Autodesk Fusion 360 part; units mm, degrees
note: some values were not read from the file. Chosen so that the rebuilt part matches the saved one: which bodies a step acts on; which sketch regions a step uses.
(part 6 of 6)
  line L3303 (-33.1167, -64.6164) -> (-31.8667, -62.4513)
  line L3304 (-48.2879, -61.8648) -> (-47.0379, -59.6997)
  line L3305 (-92.6, -56.7847) -> (-93.85, -54.6196)
  line L3306 (-20.4213, -63.2013) -> (-21.6713, -65.3664)
  line L3307 (-36.8667, -62.4513) -> (-35.6167, -64.6164)
  line L3308 (-60.9101, -61.8648) -> (-58.4101, -61.8648)
  line L3309 (-46.9889, -62.4513) -> (-45.7389, -64.6164)
  line L3310 (-35.6167, -60.2863) -> (-36.8667, -62.4513)
  line L3311 (-58.4101, -61.8648) -> (-57.1601, -59.6997)
  line L3312 (-45.7389, -64.6164) -> (-43.2389, -64.6164)
  line L3313 (-22.9944, -64.6164) -> (-21.7444, -62.4513)
  line L3314 (-30.5435, -63.2013) -> (-31.7935, -65.3664)
  line L3315 (-10.299, -63.2013) -> (-11.549, -65.3664)
  line L3316 (-58.4101, -57.5347) -> (-60.9101, -57.5347)
  line L3317 (-50.7879, -67.5315) -> (-48.2879, -67.5315)
  line L3318 (-101.399, -61.8648) -> (-98.899, -61.8648)
  line L3319 (-43.2389, -60.2863) -> (-45.7389, -60.2863)
  line L3320 (-12.8722, -64.6164) -> (-11.6222, -62.4513)
  line L3321 (-10.299, -67.5315) -> (-7.799, -67.5315)
  line L3322 (-91.2768, -61.8648) -> (-88.7768, -61.8648)
  line L3323 (-7.799, -67.5315) -> (-6.549, -65.3664)
  line L3324 (-52.0379, -65.3664) -> (-50.7879, -67.5315)
  line L3325 (-21.7444, -62.4513) -> (-22.9944, -60.2863)
  line L3326 (-26.7935, -65.3664) -> (-28.0435, -63.2013)
  line L3327 (-5.25, -64.6164) -> (-2.75, -64.6164)
  line L3328 (-20.4213, -67.5315) -> (-17.9213, -67.5315)
  line L3329 (-25.4944, -60.2863) -> (-26.7444, -62.4513)
  line L3330 (-68.5324, -57.5347) -> (-71.0324, -57.5347)
  line L3331 (-38.1657, -63.2013) -> (-40.6657, -63.2013)
  line L3332 (-1.5, -62.4513) -> (-2.75, -60.2863)
  line L3333 (-48.2879, -63.2013) -> (-50.7879, -63.2013)
  line L3334 (-43.2389, -64.6164) -> (-41.9889, -62.4513)
  line L3335 (-98.899, -61.8648) -> (-97.649, -59.6997)
  line L3336 (-6.5, -62.4513) -> (-5.25, -64.6164)
  line L3337 (-45.7389, -60.2863) -> (-46.9889, -62.4513)
  line L3338 (-30.5435, -67.5315) -> (-28.0435, -67.5315)
  line L3339 (-22.9944, -60.2863) -> (-25.4944, -60.2863)
  line L3340 (-11.6222, -62.4513) -> (-12.8722, -60.2863)
  line L3341 (-6.549, -65.3664) -> (-7.799, -63.2013)
  line L3342 (-98.899, -57.5347) -> (-101.399, -57.5347)
  line L3343 (-33.1167, -60.2863) -> (-35.6167, -60.2863)
  line L3344 (-78.6546, -61.8648) -> (-77.4046, -59.6997)
  line L3345 (-96.35, -58.9497) -> (-93.85, -58.9497)
  line L3346 (-57.1111, -56.7847) -> (-55.8611, -58.9497)
  line L3347 (-28.0435, -63.2013) -> (-30.5435, -63.2013)
  line L3348 (-97.649, -59.6997) -> (-98.899, -57.5347)
  line L3349 (-63.4833, -58.9497) -> (-62.2333, -56.7847)
  line L3350 (-41.9157, -65.3664) -> (-40.6657, -67.5315)
  line L3351 (-40.6657, -67.5315) -> (-38.1657, -67.5315)
  line L3352 (-17.9213, -67.5315) -> (-16.6713, -65.3664)
  line L3353 (-26.7444, -62.4513) -> (-25.4944, -64.6164)
  line L3354 (-15.3722, -60.2863) -> (-16.6222, -62.4513)
  line L3355 (-96.35, -54.6196) -> (-97.6, -56.7847)
  line L3356 (-15.3722, -64.6164) -> (-12.8722, -64.6164)
  line L3357 (-31.7935, -65.3664) -> (-30.5435, -67.5315)
  line L3358 (-50.7879, -63.2013) -> (-52.0379, -65.3664)
  line L3359 (-11.549, -65.3664) -> (-10.299, -67.5315)
  line L3360 (-2.75, -60.2863) -> (-5.25, -60.2863)
  line L3361 (-52.1111, -62.4513) -> (-53.3611, -60.2863)
  line L3362 (-55.8611, -60.2863) -> (-57.1111, -62.4513)
  line L3363 (-60.9101, -67.5315) -> (-58.4101, -67.5315)
  line L3364 (-91.2768, -63.2013) -> (-92.5268, -65.3664)
  line L3365 (-78.6546, -67.5315) -> (-77.4046, -65.3664)
  line L3366 (-67.2824, -65.3664) -> (-68.5324, -63.2013)
  line L3367 (-73.6056, -60.2863) -> (-76.1056, -60.2863)
  line L3368 (-68.5324, -63.2013) -> (-71.0324, -63.2013)
  line L3369 (-82.4778, -62.4513) -> (-83.7278, -60.2863)
  line L3370 (-63.4833, -60.2863) -> (-65.9833, -60.2863)
  line L3371 (-53.3611, -60.2863) -> (-55.8611, -60.2863)
  line L3372 (-7.799, -63.2013) -> (-10.299, -63.2013)
  line L3373 (-2.75, -64.6164) -> (-1.5, -62.4513)
  line L3374 (-91.2768, -67.5315) -> (-88.7768, -67.5315)
  line L3375 (-63.4833, -64.6164) -> (-62.2333, -62.4513)
  line L3376 (-76.1056, -60.2863) -> (-77.3556, -62.4513)
  line L3377 (-78.6546, -63.2013) -> (-81.1546, -63.2013)
  line L3378 (-101.399, -57.5347) -> (-102.649, -59.6997)
  line L3379 (-92.5268, -65.3664) -> (-91.2768, -67.5315)
  line L3380 (-58.4101, -63.2013) -> (-60.9101, -63.2013)
  line L3381 (-12.8722, -60.2863) -> (-15.3722, -60.2863)
  line L3382 (-5.25, -60.2863) -> (-6.5, -62.4513)
  line L3383 (-68.5324, -67.5315) -> (-67.2824, -65.3664)
  line L3384 (-87.4778, -62.4513) -> (-86.2278, -64.6164)
  line L3385 (-67.2333, -62.4513) -> (-65.9833, -64.6164)
  line L3386 (-65.9833, -60.2863) -> (-67.2333, -62.4513)
  line L3387 (-58.4101, -67.5315) -> (-57.1601, -65.3664)
  line L3388 (-86.2278, -60.2863) -> (-87.4778, -62.4513)
  line L3389 (-55.8611, -64.6164) -> (-53.3611, -64.6164)
  line L3390 (-88.7768, -63.2013) -> (-91.2768, -63.2013)
  line L3391 (-77.3556, -62.4513) -> (-76.1056, -64.6164)
  line L3392 (-71.0324, -67.5315) -> (-68.5324, -67.5315)
  line L3393 (-77.3556, -11.4513) -> (-76.1056, -13.6164)
  line L3394 (-77.4046, -65.3664) -> (-78.6546, -63.2013)
  line L3395 (-17.9213, -63.2013) -> (-20.4213, -63.2013)
  line L3396 (-73.6056, -64.6164) -> (-72.3556, -62.4513)
  line L3397 (-76.1056, -13.6164) -> (-73.6056, -13.6164)
  line L3398 (-73.6056, -13.6164) -> (-72.3556, -11.4513)
  line L3399 (-38.1657, -67.5315) -> (-36.9157, -65.3664)
  line L3400 (-86.2278, -64.6164) -> (-83.7278, -64.6164)
  line L3401 (-88.7768, -67.5315) -> (-87.5268, -65.3664)
  line L3402 (-62.2333, -62.4513) -> (-63.4833, -60.2863)
  line L3403 (-62.1601, -65.3664) -> (-60.9101, -67.5315)
  line L3404 (-72.3556, -62.4513) -> (-73.6056, -60.2863)
  line L3405 (-81.1546, -63.2013) -> (-82.4046, -65.3664)
  line L3406 (-21.6713, -65.3664) -> (-20.4213, -67.5315)
  line L3407 (-76.1056, -64.6164) -> (-73.6056, -64.6164)
  line L3408 (-57.1601, -65.3664) -> (-58.4101, -63.2013)
  line L3409 (-40.6657, -63.2013) -> (-41.9157, -65.3664)
  line L3410 (-60.9101, -63.2013) -> (-62.1601, -65.3664)
  line L3411 (-72.2824, -65.3664) -> (-71.0324, -67.5315)
  line L3412 (-81.1546, -67.5315) -> (-78.6546, -67.5315)
  line L3413 (-65.9833, -64.6164) -> (-63.4833, -64.6164)
  line L3414 (-83.7278, -60.2863) -> (-86.2278, -60.2863)
  line L3415 (-71.0324, -63.2013) -> (-72.2824, -65.3664)
  line L3416 (-57.1111, -62.4513) -> (-55.8611, -64.6164)
  line L3417 (-28.0435, -67.5315) -> (-26.7935, -65.3664)
  line L3418 (-53.3611, -64.6164) -> (-52.1111, -62.4513)
  line L3419 (-48.2879, -67.5315) -> (-47.0379, -65.3664)
  line L3420 (-82.4046, -65.3664) -> (-81.1546, -67.5315)
  line L3421 (-41.9889, -62.4513) -> (-43.2389, -60.2863)
  line L3422 (-83.7278, -64.6164) -> (-82.4778, -62.4513)
  line L3423 (-47.0379, -65.3664) -> (-48.2879, -63.2013)
  line L3424 (-25.4944, -64.6164) -> (-22.9944, -64.6164)
  line L3425 (-72.3556, -11.4513) -> (-73.6056, -9.2863)
  line L3426 (-73.6056, -9.2863) -> (-76.1056, -9.2863)
  line L3427 (-86.2278, -13.6164) -> (-83.7278, -13.6164)
  line L3428 (-81.1546, -12.2013) -> (-82.4046, -14.3664)
  line L3429 (-82.4046, -14.3664) -> (-81.1546, -16.5315)
  line L3430 (-81.1546, -16.5315) -> (-78.6546, -16.5315)
  line L3431 (-77.4046, -14.3664) -> (-78.6546, -12.2013)
  line L3432 (-87.4778, -11.4513) -> (-86.2278, -13.6164)
  line L3433 (-76.1056, -9.2863) -> (-77.3556, -11.4513)
  line L3434 (-78.6546, -12.2013) -> (-81.1546, -12.2013)
  line L3435 (-78.6546, -16.5315) -> (-77.4046, -14.3664)
  line L3436 (-83.7278, -13.6164) -> (-82.4778, -11.4513)
  line L3437 (-82.4778, -11.4513) -> (-83.7278, -9.2863)
  line L3438 (-83.7278, -9.2863) -> (-86.2278, -9.2863)
  line L3439 (-100, -76.4513) -> (0, -76.4513)
  arc A0 (-83, -31.5) -> (-81.5, -30) centre (-81.5, -31.5) cw
  line L3440 (-5.25, -77.2863) -> (-6.5, -79.4513)
  line L3441 (-7.5, -67) -> (-8.5, -67)
  arc A1 (-81.5, -67.1954) -> (-83, -65.6954) centre (-81.5, -65.6954) cw
  line L3442 (-83.3, -46.9053) -> (-88.25, -49.7631)
  line L3443 (0, -21) -> (-100, -21)
  arc A2 (-90.5, -30) -> (-89, -31.5) centre (-90.5, -31.5) cw
  line L3444 (-100, -74.4513) -> (0, -74.4513)
  line L3445 (0, -74.4513) -> (0, -21)
  arc A3 (-94, -31.5) -> (-92.5, -30) centre (-92.5, -31.5) cw
  circle A4 centre (-50, -50) radius 3.175
  arc A5 (-89, -65.5) -> (-90.5, -67) centre (-90.5, -65.5) cw
  line L3446 (-81, -67.1954) -> (-81.5, -67.1954)
  line L3447 (-90.5, -67) -> (-92.5, -67)
  line L3448 (-94, -65.5) -> (-94, -31.5)
  arc A6 (-7.5, -30) -> (-6, -31.5) centre (-7.5, -31.5) cw
  arc A7 (-83, -47.0785) -> (-83.3, -46.9053) centre (-83.2, -47.0785) ccw
  arc A8 (-83.75, -45.433) -> (-83, -44.134) centre (-84.5, -44.134) ccw
  arc A9 (-81, -30) -> (-79.5, -31.5) centre (-81, -31.5) cw
  line L3449 (-89, -51.0622) -> (-89, -65.5)
  line L3450 (-89, -31.5) -> (-89, -48.1177)
  line L3451 (-79.5, -31.5) -> (-79.5, -65.6954)
  arc A10 (-79.5, -65.6954) -> (-81, -67.1954) centre (-81, -65.6954) cw
  arc A11 (-89, -48.1177) -> (-88.7, -48.2909) centre (-88.8, -48.1177) ccw
  line L3452 (-83, -65.6954) -> (-83, -47.0785)
  arc A12 (-88.25, -49.7631) -> (-89, -51.0622) centre (-87.5, -51.0622) ccw
  line L3453 (-10, -65.5) -> (-10, -31.5)
  line L3454 (-6, -31.5) -> (-6, -65.5)
  line L3455 (-6.5, -79.4513) -> (-5.25, -81.6164)
  line L3456 (-92.5, -30) -> (-90.5, -30)
  line L3457 (-81.5, -30) -> (-81, -30)
  line L3458 (-5.25, -81.6164) -> (-2.75, -81.6164)
  line L3459 (-2.75, -77.2863) -> (-5.25, -77.2863)
  line L3460 (-8.5, -30) -> (-7.5, -30)
  line L3461 (-83, -44.134) -> (-83, -31.5)
  line L3462 (-2.75, -81.6164) -> (-1.5, -79.4513)
  line L3463 (-88.7, -48.2909) -> (-83.75, -45.433)
  arc A13 (-92.5, -67) -> (-94, -65.5) centre (-92.5, -65.5) cw
  arc A14 (-8.5, -67) -> (-10, -65.5) centre (-8.5, -65.5) cw
  line L3464 (-6.549, -3.0331) -> (-7.799, -0.868)
  line L3465 (-100, -21) -> (-100, -74.4513)
  line L3466 (-1.5, -79.4513) -> (-2.75, -77.2863)
  line L3467 (-10.299, -80.2013) -> (-11.549, -82.3664)
  line L3468 (0, -76.4513) -> (0, -84.1184)
  line L3469 (-11.6222, -0.118) -> (-12.8722, 2.0471)
  line L3470 (-36.8667, -0.118) -> (-35.6167, -2.2831)
  line L3471 (-21.7444, -0.118) -> (-22.9944, 2.0471)
  line L3472 (-7.799, -80.2013) -> (-10.299, -80.2013)
  line L3473 (-21.6713, -3.0331) -> (-20.4213, -5.1981)
  line L3474 (-33.1167, 2.0471) -> (-35.6167, 2.0471)
  line L3475 (-2.75, 2.0471) -> (-5.25, 2.0471)
  line L3476 (-11.549, -82.3664) -> (-10.299, -84.5315)
  line L3477 (-45.7389, 2.0471) -> (-46.9889, -0.118)
  line L3478 (-50.7879, -0.868) -> (-52.0379, -3.0331)
  line L3479 (-33.1167, -2.2831) -> (-31.8667, -0.118)
  line L3480 (-17.9213, -0.868) -> (-20.4213, -0.868)
  line L3481 (-12.8722, -2.2831) -> (-11.6222, -0.118)
  line L3482 (-4, -79.4513) -> (-10.924, -83.4489)
  line L3483 (-5.25, -2.2831) -> (-2.75, -2.2831)
  line L3484 (-7.799, -84.5315) -> (-6.549, -82.3664)
  line L3485 (-20.4213, -5.1981) -> (-17.9213, -5.1981)
  line L3486 (-40.6657, -5.1981) -> (-38.1657, -5.1981)
  line L3487 (-41.9889, -0.118) -> (-43.2389, 2.0471)
  line L3488 (-31.8667, -0.118) -> (-33.1167, 2.0471)
  line L3489 (-6.549, -82.3664) -> (-7.799, -80.2013)
  line L3490 (-17.9213, -5.1981) -> (-16.6713, -3.0331)
  line L3491 (-28.0435, -5.1981) -> (-26.7935, -3.0331)
  line L3492 (-40.6657, -0.868) -> (-41.9157, -3.0331)
  arc A15 (-6, -65.5) -> (-7.5, -67) centre (-7.5, -65.5) cw
  line L3493 (-30.5435, -5.1981) -> (-28.0435, -5.1981)
  line L3494 (-26.7935, -3.0331) -> (-28.0435, -0.868)
  line L3495 (-43.2389, -2.2831) -> (-41.9889, -0.118)
  line L3496 (-16.6713, -3.0331) -> (-17.9213, -0.868)
  arc A16 (-10, -31.5) -> (-8.5, -30) centre (-8.5, -31.5) cw
  line L3497 (-43.2389, 2.0471) -> (-45.7389, 2.0471)
  line L3498 (-28.0435, -0.868) -> (-30.5435, -0.868)
  line L3499 (-5.25, 2.0471) -> (-6.5, -0.118)
  line L3500 (-41.9157, -3.0331) -> (-40.6657, -5.1981)
  line L3501 (-52.0379, -3.0331) -> (-50.7879, -5.1981)
  line L3502 (-31.7935, -3.0331) -> (-30.5435, -5.1981)
  line L3503 (-48.2879, -0.868) -> (-50.7879, -0.868)
  line L3504 (-50.7879, -5.1981) -> (-48.2879, -5.1981)
  line L3505 (-20.4213, -0.868) -> (-21.6713, -3.0331)
  line L3506 (-30.5435, -0.868) -> (-31.7935, -3.0331)
  line L3507 (-22.9944, -2.2831) -> (-21.7444, -0.118)
  line L3508 (-10.299, -5.1981) -> (-7.799, -5.1981)
  line L3509 (-45.7389, -2.2831) -> (-43.2389, -2.2831)
  line L3510 (-6.5, -0.118) -> (-5.25, -2.2831)
  line L3511 (-7.799, -5.1981) -> (-6.549, -3.0331)
  line L3512 (-2.75, -2.2831) -> (-1.5, -0.118)
  line L3513 (-26.7444, -0.118) -> (-25.4944, -2.2831)
  line L3514 (-15.3722, -2.2831) -> (-12.8722, -2.2831)
  line L3515 (-35.6167, 2.0471) -> (-36.8667, -0.118)
  line L3516 (-11.549, -3.0331) -> (-10.299, -5.1981)
  line L3517 (-15.3722, 2.0471) -> (-16.6222, -0.118)
  line L3518 (-73.6056, 2.0471) -> (-76.1056, 2.0471)
  line L3519 (-65.9833, -2.2831) -> (-63.4833, -2.2831)
  line L3520 (-25.4944, 2.0471) -> (-26.7444, -0.118)
  line L3521 (-86.2278, 2.0471) -> (-87.4778, -0.118)
  line L3522 (-72.2824, -3.0331) -> (-71.0324, -5.1981)
  line L3523 (-91.2768, -0.868) -> (-92.5268, -3.0331)
  line L3524 (-93.85, -2.2831) -> (-92.6, -0.118)
  line L3525 (-35.6167, -2.2831) -> (-33.1167, -2.2831)
  line L3526 (-46.9889, -0.118) -> (-45.7389, -2.2831)
  line L3527 (-38.1657, -5.1981) -> (-36.9157, -3.0331)
  line L3528 (-1.5, -0.118) -> (-2.75, 2.0471)
  line L3529 (-10.299, -84.5315) -> (-7.799, -84.5315)
  line L3530 (-55.8611, 2.0471) -> (-57.1111, -0.118)
  line L3531 (-92.6, -0.118) -> (-93.85, 2.0471)
  line L3532 (-96.35, 2.0471) -> (-97.6, -0.118)
  line L3533 (-38.1657, -0.868) -> (-40.6657, -0.868)
  line L3534 (-96.35, -2.2831) -> (-93.85, -2.2831)
  line L3535 (-12.8722, 2.0471) -> (-15.3722, 2.0471)
  line L3536 (-36.9157, -3.0331) -> (-38.1657, -0.868)
  line L3537 (-16.6222, -0.118) -> (-15.3722, -2.2831)
  line L3538 (-7.799, -0.868) -> (-10.299, -0.868)
  line L3539 (-71.0324, -5.1981) -> (-68.5324, -5.1981)
  line L3540 (-101.399, -0.868) -> (-102.649, -3.0331)
  line L3541 (-57.1601, -3.0331) -> (-58.4101, -0.868)
  line L3542 (-22.9944, 2.0471) -> (-25.4944, 2.0471)
  line L3543 (-10.299, -0.868) -> (-11.549, -3.0331)
  line L3544 (-25.4944, -2.2831) -> (-22.9944, -2.2831)
  line L3545 (-53.3611, -2.2831) -> (-52.1111, -0.118)
  line L3546 (-86.2278, -2.2831) -> (-83.7278, -2.2831)
  line L3547 (-77.3556, -0.118) -> (-76.1056, -2.2831)
  line L3548 (-67.2824, -3.0331) -> (-68.5324, -0.868)
  line L3549 (-71.0324, -0.868) -> (-72.2824, -3.0331)
  line L3550 (-48.2879, -5.1981) -> (-47.0379, -3.0331)
  line L3551 (-98.899, -5.1981) -> (-97.649, -3.0331)
  line L3552 (-83.7278, -2.2831) -> (-82.4778, -0.118)
  line L3553 (-102.649, -3.0331) -> (-101.399, -5.1981)
  line L3554 (-62.2333, -0.118) -> (-63.4833, 2.0471)
  line L3555 (-43.2389, -71.6196) -> (-45.7389, -71.6196)
  line L3556 (-45.7389, -71.6196) -> (-46.9889, -73.7847)
  line L3557 (-50.7879, -74.5347) -> (-52.0379, -76.6997)
  line L3558 (-48.2879, -74.5347) -> (-50.7879, -74.5347)
  line L3559 (-52.0379, -76.6997) -> (-50.7879, -78.8648)
  line L3560 (-45.7389, -65.9529) -> (-46.9889, -68.118)
  line L3561 (-43.2389, -65.9529) -> (-45.7389, -65.9529)
  line L3562 (-41.9889, -68.118) -> (-43.2389, -65.9529)
  line L3563 (-48.2879, -73.1981) -> (-47.0379, -71.0331)
  line L3564 (-50.7879, -73.1981) -> (-48.2879, -73.1981)
  line L3565 (-47.0379, -71.0331) -> (-48.2879, -68.868)
  line L3566 (-57.1111, -68.118) -> (-55.8611, -70.2831)
  line L3567 (-53.3611, -70.2831) -> (-52.1111, -68.118)
  line L3568 (-52.0379, -71.0331) -> (-50.7879, -73.1981)
  line L3569 (-50.7879, -78.8648) -> (-48.2879, -78.8648)
  line L3570 (-50.7879, -68.868) -> (-52.0379, -71.0331)
  line L3571 (-55.8611, -65.9529) -> (-57.1111, -68.118)
  line L3572 (-63.4833, -70.2831) -> (-62.2333, -68.118)
  line L3573 (-65.9833, -65.9529) -> (-67.2333, -68.118)
  line L3574 (-81.1546, -68.868) -> (-82.4046, -71.0331)
  line L3575 (-73.6056, -70.2831) -> (-72.3556, -68.118)
  line L3576 (-87.4778, -68.118) -> (-86.2278, -70.2831)
  line L3577 (-68.5324, -68.868) -> (-71.0324, -68.868)
  line L3578 (-58.4101, -68.868) -> (-60.9101, -68.868)
  line L3579 (-93.85, -70.2831) -> (-92.6, -68.118)
  line L3580 (-60.9101, -73.1981) -> (-58.4101, -73.1981)
  line L3581 (-68.5324, -73.1981) -> (-67.2824, -71.0331)
  line L3582 (-92.5268, -71.0331) -> (-91.2768, -73.1981)
  line L3583 (-76.1056, -70.2831) -> (-73.6056, -70.2831)
  line L3584 (-73.6056, -65.9529) -> (-76.1056, -65.9529)
  line L3585 (-92.6, -68.118) -> (-93.85, -65.9529)
  line L3586 (-72.3556, -68.118) -> (-73.6056, -65.9529)
  line L3587 (-58.4101, -73.1981) -> (-57.1601, -71.0331)
  line L3588 (-72.2824, -71.0331) -> (-71.0324, -73.1981)
  line L3589 (-86.2278, -70.2831) -> (-83.7278, -70.2831)
  line L3590 (-65.9833, -70.2831) -> (-63.4833, -70.2831)
  line L3591 (-62.1601, -71.0331) -> (-60.9101, -73.1981)
  line L3592 (-62.2333, -68.118) -> (-63.4833, -65.9529)
  line L3593 (-67.2824, -71.0331) -> (-68.5324, -68.868)
  line L3594 (-91.2768, -73.1981) -> (-88.7768, -73.1981)
  line L3595 (-76.1056, -65.9529) -> (-77.3556, -68.118)
  line L3596 (-52.1111, -68.118) -> (-53.3611, -65.9529)
  line L3597 (-83.7278, -70.2831) -> (-82.4778, -68.118)
  line L3598 (-83.7278, -65.9529) -> (-86.2278, -65.9529)
  line L3599 (-88.7768, -68.868) -> (-91.2768, -68.868)
  line L3600 (-96.35, -70.2831) -> (-93.85, -70.2831)
  line L3601 (-78.6546, -68.868) -> (-81.1546, -68.868)
  line L3602 (-91.2768, -68.868) -> (-92.5268, -71.0331)
  line L3603 (-93.85, -65.9529) -> (-96.35, -65.9529)
  line L3604 (-60.9101, -68.868) -> (-62.1601, -71.0331)
  line L3605 (-71.0324, -73.1981) -> (-68.5324, -73.1981)
  line L3606 (-82.4778, -68.118) -> (-83.7278, -65.9529)
  line L3607 (-77.4046, -71.0331) -> (-78.6546, -68.868)
  line L3608 (-55.8611, -70.2831) -> (-53.3611, -70.2831)
  line L3609 (-96.35, -65.9529) -> (-97.6, -68.118)
  line L3610 (-101.399, -68.868) -> (-102.649, -71.0331)
  line L3611 (-82.4046, -71.0331) -> (-81.1546, -73.1981)
  line L3612 (-67.2333, -68.118) -> (-65.9833, -70.2831)
  line L3613 (-63.4833, -65.9529) -> (-65.9833, -65.9529)
  line L3614 (-86.2278, -65.9529) -> (-87.4778, -68.118)
  line L3615 (-77.3556, -68.118) -> (-76.1056, -70.2831)
  line L3616 (-102.649, -71.0331) -> (-101.399, -73.1981)
  line L3617 (-71.0324, -68.868) -> (-72.2824, -71.0331)
  line L3618 (-48.2879, -68.868) -> (-50.7879, -68.868)
  line L3619 (-57.1601, -71.0331) -> (-58.4101, -68.868)
  line L3620 (-81.1546, -73.1981) -> (-78.6546, -73.1981)
  line L3621 (-78.6546, -73.1981) -> (-77.4046, -71.0331)
  line L3622 (-53.3611, -65.9529) -> (-55.8611, -65.9529)
extrude "Extrude22" cut sketch "holes" against normal up to surface (2.5 mm away) contours L0 L9 L26 L27 L40 L43 | L3 L10 L11 L33 L48 L54 | L4 L15 L28 L35 L55 L120 | L5 L6 L17 L39 L47 L123 | L12 L14 L25 L32 L42 L126 | L13 L16 L22 L31 L41 L45 | L19 L20 L21 L24 L121 L125 | L56 L73 L76 L83 L87 L1162 | L57 L60 L69 L77 L103 L109 | L59 L72 L84 L92 L104 L111 | L63 L64 L78 L90 L105 L113 | L70 L85 L88 L97 L106 L114 | L95 L100 L101 L110 L1161 L1174 | L333 L336 L354 L355 L371 L397 | L422 L423 L424 L438 L485 L532 | L435 L453 L459 L472 L489 L503 | L457 L463 L464 L480 L498 L505 | L460 L471 L486 L501 L519 L533 | L461 L474 L476 L478 L499 L506 | L467 L481 L488 L492 L513 L541 | L509 L515 L523 L531 L543 L544 | L512 L542 L546 L554 L555 L566 | L516 L518 L520 L521 L529 L536 | L550 L556 L557 L559 L568 L573 | L1008 L1014 L1015 L1042 L1054 L1177 | L1009 L1028 L1030 L1037 L1044 L1166 | L1010 L1018 L1019 L1020 L1045 L1164 | L1016 L1017 L1029 L1034 L1052 L1179 | L1021 L1022 L1024 L1031 L1032 L1171 | L1025 L1035 L1038 L1048 L1169 L1176 | L1026 L1027 L1049 L1056 L1160 L1163 | L1033 L1041 L1046 L1165 L1175 L1178 | L1040 L1047 L1158 L1159 L1167 L1168 | L1050 L1057 L1058 L1110 L1113 L1117 | L1055 L1059 L1075 L1088 L1106 L1114 | L1060 L1061 L1079 L1080 L1103 L1124 | L1062 L1072 L1083 L1084 L1100 L1120 | L1063 L1074 L1077 L1090 L1099 L1105 | L1064 L1081 L1082 L1087 L1098 L1132 | L1066 L1076 L1085 L1093 L1102 L1104 | L1070 L1073 L1078 L1096 L1107 L1115 | L1071 L1086 L1091 L1095 L1135 L1142 | L1108 L1109 L1128 L1131 L1144 L1200 | L1111 L1121 L1123 L1136 L1182 L1237 | L1112 L1133 L1141 L1155 L1213 L1228 | L1116 L1134 L1143 L1156 L1193 L1204 | L1118 L1140 L1185 L1192 L1195 L1243 | L1119 L1138 L1148 L1201 L1225 L1233 | L1122 L1129 L1130 L1153 L1191 L1198 | L1126 L1127 L1151 L1152 L1207 L1236 | L1137 L1139 L1145 L1146 L1147 L1149 | L1150 L1154 L1157 L1197 L1202 L1226 | L1181 L1205 L1216 L1217 L1227 L1241 | L1183 L1187 L1208 L1220 L1230 L1234 | L1184 L1189 L1194 L1206 L1238 L1260 | L1186 L1199 L1212 L1218 L1252 L1261 | L1190 L1219 L1221 L1231 L1240 L1265 | L1196 L1242 L1248 L1254 L1258 L1280 | L1203 L1222 L1249 L1285 L1295 L1307 | L1211 L1224 L1247 L1262 L1267 L1286 | L1244 L1290 L1306 L1324 L1332 L1352 | L1245 L1251 L1259 L1270 L1294 L1299 | L1246 L1264 L1312 L1321 L1353 L1361 | L1250 L1274 L1279 L1346 L1351 L1359 | L1253 L1276 L1292 L1298 L1303 L1360 | L1255 L1269 L1287 L1338 L1340 L1347 | L1256 L1268 L1281 L1283 L1284 L1337 | L1257 L1282 L1300 L1302 L1304 L1348 | L1263 L1291 L1301 L1305 L1316 L1371 | L1266 L1296 L1315 L1331 L1336 L1357 | L1271 L1272 L1278 L1288 L1289 L1349 | L1273 L1275 L1277 L1297 L1342 L1367 | L1308 L1314 L1369 L1377 L1395 L1431 | L1309 L1319 L1339 L1355 L1358 L1368 | L1310 L1374 L1384 L1397 L1402 L1423 | L1311 L1320 L1327 L1333 L1334 L1387 | L1313 L1356 L1362 L1366 L1382 L1394 | L1318 L1326 L1329 L1330 L1343 L1389 | L1322 L1323 L1364 L1383 L1399 L1418 | L1341 L1344 L1350 L1363 L1370 L1405 | L1345 L1379 L1409 L1435 L1458 L1476 | L1375 L1407 L1408 L1413 L1446 L1469 | L1376 L1398 L1403 L1406 L1460 L1482 | L1378 L1415 L1429 L1461 L1492 L1493 | L1380 L1386 L1426 L1432 L1450 L1471 | L1381 L1390 L1416 L1440 L1474 L1491 | L1385 L1412 L1427 L1428 L1456 L1459 | L1391 L1421 L1437 L1472 L1483 L1489 | L1400 L1401 L1410 L1433 L1434 L1495 | L1417 L1419 L1420 L1424 L1430 L1473 | L1436 L1486 L1497 L1530 L1533 L1556 | L1438 L1444 L1448 L1463 L1470 L1481 | L1441 L1467 L1468 L1524 L1553 L1560 | L1442 L1496 L1512 L1517 L1539 L1557 | L1445 L1465 L1477 L1479 L1488 L1499 | L1447 L1455 L1494 L1498 L1505 L1510 | L1452 L1478 L1480 L1501 L1522 L1624 | L1457 L1475 L1490 L1502 L1520 L1548 | L1503 L1504 L1558 L1573 L1575 L1588 | L1506 L1514 L1541 L1554 L1587 L1592 | L1507 L1509 L1544 L1607 L1612 L1613 | L1528 L1549 L1559 L1585 L1604 L1620 | L1529 L1552 L1555 L1561 L1574 L1602 | L1568 L1579 L1595 L1623 L1641 L1648 | L1569 L1580 L1626 L1627 L1649 L1667 | L1590 L1594 L1611 L1617 L1621 L1639 | L1597 L1618 L1646 L1655 L1681 L1688 | L1631 L1634 L1658 L1692 L1714 L1716 | L1638 L1651 L1654 L1669 L1672 L1689 bodies 5
fillet "Fillet11" radius 12.5 2 edges at (140.0889, 171.2251, 1.25) (260.0889, 171.2251, 1.25) on bodies 5
fillet "Fillet12" radius 10 1 edges at (139.9111, 114.4436, 1.25) on bodies 5
fillet "Fillet13" radius 10 1 edges at (260.0889, 114.4436, 1.25) on bodies 5
fillet "Fillet14" radius 10 1 edges at (200.0889, 152.2502, 1.25) on bodies 5
fillet "Fillet15" radius 10 1 edges at (200.0889, 121.2181, 1.25) on bodies 5
equation "d12 = 4 mm + 3.1 mm"
equation "d14 = 31.35 mm + 6.2 mm"
equation "d17 = 31.35 mm + 6.2 mm"
equation "d24 = ( ( 50 - 35 ) / 2 ) * 1 mm"
equation "d55 = ( 45 / 2 ) * 1 mm"
equation "d58 = -4 mm + -4 mm + -2.5 mm"
equation "d63 = ( 35 / 2 ) * 1 mm"
